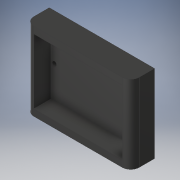
# Autodesk Inventor part: BatteryHolder
Saved by Autodesk Inventor 2018 (Build 220112000, 112)
## iProperties
Created: 2018-01-13
Part Number: BatteryHolder
Material: ABS Plastic
Document SubType Name: Modeling
Designer: Kyle-HP
Density: 1.06 g/cm^3
Appearance: Smooth - Black
Author: Kyle-HP
Autodesk Inventor part; units mm, degrees
ref_plane "YZ Plane" through (0, 0, 0) normal (1, 0, 0) x (0, 1, 0)
ref_plane "XZ Plane" through (0, 0, 0) normal (0, 1, 0) x (-1, 0, 0)
ref_plane "XY Plane" through (0, 0, 0) normal (0, 0, 1) x (1, 0, 0)
sketch "Sketch1" plane through (0, 0, 0) normal (0, 0, 1) x (1, 0, 0)
  line L0 (0, 0) -> (78.74, 0)
  line L1 (78.74, 0) -> (78.74, -58.42)
  line L2 (78.74, -58.42) -> (0, -58.42)
  line L3 (0, -58.42) -> (0, 0)
  dimension "d0" = 78.74
  dimension "d1" = 58.42
  constraints: 8 end point, 2 parallel, 1 horizontal, 1 perpendicular
  measures "d0" distance of L0.start L0.end
  measures "d1" distance of L2.end L0.start
extrude "Extrusion1" add sketch "Sketch1" along normal blind 17.78
fillet "Fillet1" radius 6.35 2 edges at (78.74, -29.21, 17.78) (0, -29.21, 17.78)
sketch "Sketch2" plane through (0, 0, 0) normal (0, 0, -1) x (-1, 0, 0)
  circle A0 centre (-69.85, -29.21) radius 1.5875
  line L0 (-78.74, 0) -> (-78.74, -58.42) projected
  line L1 (0, 0) -> (-78.74, 0) projected
  circle A1 centre (-8.89, -29.21) radius 1.5875
  line L2 (0, -58.42) -> (0, 0) projected
  dimension "d5" = 3.175
  dimension "d6" = 8.89
  dimension "d7" = 29.21
  dimension "d8" = 3.175
  dimension "d9" = 8.89
  constraints: 2 centre point
  measures "d5" diameter of A0
  measures "d6" distance from line of L0 A0.centre
  measures "d7" distance from line of A0.centre L1
  measures "d8" diameter of A1
  measures "d9" distance from line of L2 A1.centre
extrude "Extrusion2" cut sketch "Sketch2" against normal blind 25.4
sketch "Sketch3" plane through (0, 0, 17.78) normal (0, 0, 1) x (1, 0, 0)
  line L0 (6.35, -58.42) -> (6.35, 0) projected
  line L1 (72.39, 0) -> (72.39, -58.42) projected
  line L2 (6.35, -5.08) -> (72.39, -5.08)
  line L3 (72.39, -5.08) -> (72.39, -53.34)
  line L4 (72.39, -53.34) -> (6.35, -53.34)
  line L5 (6.35, -53.34) -> (6.35, -5.08)
  line L6 (72.39, 0) -> (6.35, 0) projected
  line L7 (6.35, -58.42) -> (72.39, -58.42) projected
  point P0 (0, 0)
  dimension "d12" = 5.08
  dimension "d13" = 5.08
  constraints: 8 end point, 2 parallel, 2 point on line, 1 horizontal, 1 perpendicular
  measures "d12" distance between parallel lines of L6 L2
  measures "d13" distance between parallel lines of L7 L4
extrude "Extrusion3" cut sketch "Sketch3" against normal blind 12.7 contours L0 L2 L1 L4
body "Solid1"
